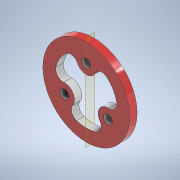
# Autodesk Inventor part: socket_extension
Saved by Autodesk Inventor 2021 (Build 250183000, 183)
## iProperties
Created: 2021-05-31
Part Number: socket_extension
Material: Generic
Document SubType Name: Modeling
Designer: ztjona!
Density: 1 g/cm^3
Appearance: Default
Author: ztjona!
Autodesk Inventor part; units mm, degrees
ref_plane "XZ Plane" through (0, 0, 0) normal (0, 1, 0) x (-1, 0, 0)
ref_plane "XY Plane" through (0, 0, 0) normal (0, 0, 1) x (1, 0, 0)
ref_plane "Work Plane1" through (0, 0, 0) normal (0, 0, 1) x (1, 0, 0)
sketch "Sketch1" plane through (0, 0, 0) normal (0, 0, 1) x (1, 0, 0)
  arc A0 (-3.6093, -0.9175) -> (-8.311, 0.0303) centre (-6.3164, -2.2106) ccw projected
  arc A1 (-3.6093, -0.9175) -> (3.6093, -0.9175) centre (0, 0.8066) ccw projected
  arc A2 (8.311, 0.0303) -> (3.6093, -0.9175) centre (6.3164, -2.2106) ccw projected
  arc A3 (12.2415, -6.7775) -> (8.311, 0.0303) centre (0, -9.3066) ccw projected
  arc A4 (9.0699, -10.3754) -> (12.2415, -6.7775) centre (9.3035, -7.3845) ccw projected
  arc A5 (9.0699, -10.3754) -> (5.4605, -16.627) centre (8.7583, -14.3632) ccw projected
  arc A6 (3.9305, -21.1726) -> (5.4605, -16.627) centre (2.9872, -18.3248) ccw projected
  arc A7 (-3.9305, -21.1726) -> (3.9305, -21.1726) centre (0, -9.3066) ccw projected
  arc A8 (-5.4605, -16.627) -> (-3.9305, -21.1726) centre (-2.9872, -18.3248) ccw projected
  arc A9 (-5.4605, -16.627) -> (-9.0699, -10.3754) centre (-8.7583, -14.3632) ccw projected
  arc A10 (-12.2415, -6.7775) -> (-9.0699, -10.3754) centre (-9.3035, -7.3845) ccw projected
  arc A11 (-8.311, 0.0303) -> (-12.2415, -6.7775) centre (0, -9.3066) ccw projected
  line L0 (-11.2583, -15.8066) -> (-8.7583, -17.25) projected
  line L1 (-11.2583, -12.9199) -> (-11.2583, -15.8066) projected
  line L2 (-8.7583, -11.4765) -> (-11.2583, -12.9199) projected
  line L3 (-6.2583, -12.9199) -> (-8.7583, -11.4765) projected
  line L4 (-6.2583, -15.8066) -> (-6.2583, -12.9199) projected
  line L5 (-8.7583, -17.25) -> (-6.2583, -15.8066) projected
  line L6 (11.2583, -15.8066) -> (11.2583, -12.9199) projected
  line L7 (8.7583, -17.25) -> (11.2583, -15.8066) projected
  line L8 (6.2583, -15.8066) -> (8.7583, -17.25) projected
  line L9 (6.2583, -12.9199) -> (6.2583, -15.8066) projected
  line L10 (8.7583, -11.4765) -> (6.2583, -12.9199) projected
  line L11 (11.2583, -12.9199) -> (8.7583, -11.4765) projected
  circle A12 centre (0, -9.3066) radius 17.5 projected
  line L12 (0, 3.6934) -> (-2.5, 2.25) projected
  line L13 (2.5, 2.25) -> (0, 3.6934) projected
  line L14 (2.5, -0.6368) -> (2.5, 2.25) projected
  line L15 (0, -2.0801) -> (2.5, -0.6368) projected
  line L16 (-2.5, -0.6368) -> (0, -2.0801) projected
  line L17 (-2.5, 2.25) -> (-2.5, -0.6368) projected
  circle A13 centre (-8.7583, -14.3632) radius 1.75
  circle A14 centre (8.7583, -14.3632) radius 1.75
  circle A15 centre (0, 0.8066) radius 1.75
  point P0 (0, 0)
  dimension "d2" = 3.5
  dimension "d3" = 3.5
  dimension "d4" = 3.5
  constraints: 3 centre point, 3 coincident
  measures "d2" diameter of A14
  measures "d3" diameter of A15
  measures "d4" diameter of A13
extrude "Extrusion1" add sketch "Sketch1" along normal blind 3 contours L1 L2 L3 L4 L5 L0 | L7 L8 L9 L10 L11 L6 | A12 | L13 L14 L15 L16 L17 L12
body "Solid1"
